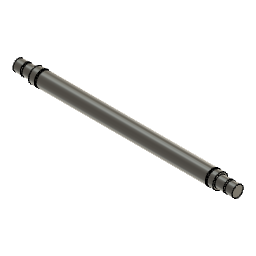
shaft (Autodesk Fusion 360 design; units mm, degrees)
Autodesk Fusion 360 part; units mm, degrees
sketch "Sketch1" plane through (0, 0, 0) normal (1, 0, 0) x (0, 1, 0)
  circle A0 centre (0, 0) radius 3
  dimension "d1" = 6
  constraint coincident A0.centre origin
  measures "d1" diameter of A0
extrude "Extrude1" add sketch "Sketch1" along normal blind 8
sketch "Sketch2" plane through (8, 0, 0) normal (1, 0, 0) x (0, 1, 0)
  circle A0 centre (0, 0) radius 3
  circle A1 centre (0, 0) radius 4
  dimension "d4" = 8
  constraint concentric A0 A1
  measures "d4" diameter of A1
extrude "Extrude2" add sketch "Sketch2" along normal blind 3.15 contours A0 | A1
sketch "Sketch3" plane through (11.15, 0, 0) normal (1, 0, 0) x (0, 1, 0)
  circle A0 centre (0, 0) radius 4
  circle A1 centre (0, 0) radius 3.775
  dimension "d7" = 7.55
  constraint concentric A0 A1
  measures "d7" diameter of A1
extrude "Extrude3" add sketch "Sketch3" along normal blind 0.85 contours A1
sketch "Sketch4" plane through (12, 0, 0) normal (1, 0, 0) x (0, 1, 0)
  circle A0 centre (0, 0) radius 3.775
  circle A1 centre (0, 0) radius 4
  dimension "d10" = 8
  constraint concentric A0 A1
  measures "d10" diameter of A1
extrude "Extrude4" add sketch "Sketch4" along normal blind 92 contours A0 | A1
sketch "Sketch5" plane through (104, 0, 0) normal (1, 0, 0) x (0, 1, 0)
  circle A0 centre (0, 0) radius 4
  circle A1 centre (0, 0) radius 3.775
  dimension "d13" = 7.55
  constraint concentric A0 A1
  measures "d13" diameter of A1
extrude "Extrude5" add sketch "Sketch5" along normal blind 0.85 contours A1
sketch "Sketch6" plane through (104.85, 0, 0) normal (1, 0, 0) x (0, 1, 0)
  circle A0 centre (0, 0) radius 3.775
  circle A1 centre (0, 0) radius 4
  dimension "d16" = 8
  constraint concentric A0 A1
  measures "d16" diameter of A1
extrude "Extrude6" add sketch "Sketch6" along normal blind 3.15 contours A0 | A1
extrude "Extrude8" cut 1 faces at (0, -1.1591, 0.5829) along direction (1, 0, 0) blind 8
sketch "Sketch8" plane through (8, 0, 0) normal (-1, 0, 0) x (0, -1, 0)
  circle A0 centre (0, 0) radius 4
  circle A1 centre (0, 0) radius 3
  dimension "d24" = 6
  constraint concentric A0 A1
  measures "d24" diameter of A1
extrude "Extrude9" add sketch "Sketch8" along normal blind 4.72 contours A1
sketch "Sketch9" plane through (3.28, 0, 0) normal (-1, 0, 0) x (0, -1, 0)
  circle A0 centre (0, 0) radius 3
  circle A1 centre (0, 0) radius 2
  dimension "d27" = 4
  constraint coincident A0.centre A1.centre
  measures "d27" diameter of A1
extrude "Extrude10" add sketch "Sketch9" along normal blind 0.75 contours A1
sketch "Sketch10" plane through (2.53, 0, 0) normal (-1, 0, 0) x (0, -1, 0)
  circle A0 centre (0, 0) radius 2
  circle A1 centre (0, 0) radius 3
  dimension "d30" = 6
  constraint concentric A0 A1
  measures "d30" diameter of A1
extrude "Extrude11" add sketch "Sketch10" along normal blind 4 contours A0 | A1
sketch "Sketch11" plane through (108, 0, 0) normal (1, 0, 0) x (0, 1, 0)
  circle A0 centre (0, 0) radius 4
  circle A1 centre (0, 0) radius 3
  dimension "d33" = 6
  constraint coincident A0.centre A1.centre
  measures "d33" diameter of A1
extrude "Extrude12" add sketch "Sketch11" along normal blind 4.72 contours A1
sketch "Sketch12" plane through (112.72, 0, 0) normal (1, 0, 0) x (0, 1, 0)
  circle A0 centre (0, 0) radius 3
  circle A1 centre (0, 0) radius 2
  dimension "d36" = 4
  constraint concentric A0 A1
  measures "d36" diameter of A1
extrude "Extrude13" add sketch "Sketch12" along normal blind 0.75 contours A1
sketch "Sketch13" plane through (113.47, 0, 0) normal (1, 0, 0) x (0, 1, 0)
  circle A0 centre (0, 0) radius 2
  circle A1 centre (0, 0) radius 3
  dimension "d39" = 6
  constraint concentric A0 A1
  measures "d39" diameter of A1
extrude "Extrude14" add sketch "Sketch13" along normal blind 4 contours A0 | A1
equation "d17 = 100 mm - 96.85 mm"
